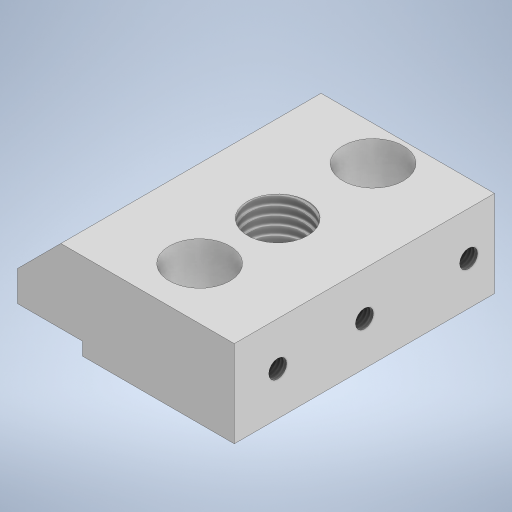
# Autodesk Inventor part: spannbakce
Saved by Autodesk Inventor 2024 (Build 280153000, 153)
## iProperties
Created: 2024-01-30
Part Number: spannbakce
Material: Generisch
Document SubType Name: Modeling
Designer: ffogue
Density: 1 g/cm^3
Appearance: Vorgabe
Author: ffogue
Autodesk Inventor part; units mm, degrees
note: some values were not read from the file. Chosen so that the rebuilt part matches the saved one: direction of "Bohrung2"; direction of "Bohrung3".
ref_plane "YZ Plane" through (0, 0, 0) normal (1, 0, 0) x (0, 1, 0)
ref_plane "XZ Plane" through (0, 0, 0) normal (0, 1, 0) x (-1, 0, 0)
ref_plane "XY Plane" through (0, 0, 0) normal (0, 0, 1) x (1, 0, 0)
sketch "Skizze1" plane through (0, 0, 0) normal (0, 1, 0) x (-1, 0, 0)
  line L0 (0, -10) -> (0, 10)
  line L1 (0, 10) -> (40, 10)
  line L2 (40, 10) -> (50, 0)
  line L3 (50, 0) -> (50, -7)
  line L4 (50, -7) -> (35, -7)
  line L5 (35, -7) -> (35, -10)
  line L6 (35, -10) -> (0, -10)
  line L7 (0, 0) -> (85.3703, 0) construction
  dimension "d0" = 10
  dimension "d1" = 10
  dimension "d2" = 3
  dimension "d3" = 20
  dimension "d4" = 40
  dimension "d5" = 15
  constraints: 17 end point, 5 perpendicular, 1 coincident, 1 horizontal, 1 midpoint, 1 vertical
  measures "d0" horizontal distance of L2.end L1.end
  measures "d1" horizontal distance of L2.end L1.end
  measures "d2" distance between parallel lines of L6 L4
  measures "d3" distance between parallel lines of L6 L1
  measures "d4" distance from line of L0 L1.end
  measures "d5" distance between parallel lines of L5 L3
extrude "Extrusion1" add sketch "Skizze1" along normal blind 60
sketch "Skizze2" plane through (-35, 0, -7) normal (0, 0, -1) x (-1, 0, 0)
  line L0 (15, 0) -> (15, 60) projected
  line L1 (15, 30) -> (5.3736, 30) construction
  line L2 (0, 60) -> (15, 60) projected
  point P0 (-35, 0)
  point P1 (8, 10)
  point P2 (8, 50)
  dimension "d8" = 7
  dimension "d9" = 7
  dimension "d10" = 40
  dimension "d11" = 10
  constraints: 2 end point, 1 horizontal, 1 midpoint
  measures "d8" distance from line of L0 point (8, 10)
  measures "d9" distance from line of point (8, 50) L0
  measures "d10" distance of point (8, 10) point (8, 50)
  measures "d11" distance from line of point (8, 50) L2
hole "Bohrung1" at (-43, 10, -7) at (-43, 50, -7) direction (0, 0, 1) diameter 3.242 depth 12 tip angle 118 thread size "M4x0.7" class "6H" standard "ISO Metric profile"
sketch "Skizze3" plane through (0, 0, -10) normal (0, 0, -1) x (-1, 0, 0)
  line L0 (0, 0) -> (0, 60) projected
  line L1 (0, 0) -> (35, 0) projected
  point P0 (20, 52)
  point P1 (20, 30)
  point P2 (20, 12)
  point P3 (0, 30)
  dimension "d19" = 20
  dimension "d20" = 12
  dimension "d21" = 40
  constraints: 3 vertical alignment, 1 horizontal alignment, 1 midpoint
  measures "d19" distance from line of L0 point (20, 52)
  measures "d20" distance from line of L1 point (20, 12)
  measures "d21" distance of point (20, 12) point (20, 52)
hole "Bohrung2" at (-20, 12, -10) at (-20, 52, -10) direction (0, 0, 1) diameter 14 depth 20
hole "Bohrung3" at (-20, 30, -10) direction (0, 0, 1) diameter 13.835 depth 20 thread size "M16x2" class "6H" standard "ISO Metric profile"
sketch "Skizze6" plane through (0, 0, 10) normal (1, 0, 0) x (0, 0, -1)
  line L0 (0, 60) -> (20, 60) projected
  point P0 (10, 0)
  point P1 (10, 54.0188)
  point P2 (10, 60)
  constraints: 1 midpoint, 1 vertical alignment
hole "Bohrung4" at (0, 54.0188, 0) direction (-1, 0, 0) diameter 4.134 depth 10 tip angle 118 thread size "M5x0.8" class "6H" standard "ISO Metric profile"
sketch "Skizze7" plane through (0, 0, 10) normal (1, 0, 0) x (0, 0, -1)
  line L0 (0, 0) -> (20, 0) projected
  point P0 (10, 0)
  point P1 (10, 10)
  point P2 (10, 0)
  point P3 (10, 0)
  dimension "d51" = 10
  constraints: 2 midpoint, 1 vertical alignment
  measures "d51" distance of point (10, 0) point (10, 10)
hole "Bohrung5" at (0, 10, 0) direction (-1, 0, 0) diameter 4.134 depth 10 tip angle 118 thread size "M5x0.8" class "6H" standard "ISO Metric profile"
sketch "Skizze8" plane through (0, 0, 10) normal (1, 0, 0) x (0, 0, -1)
  line L0 (0, 0) -> (20, 0) projected
  point P0 (10, 0)
  point P1 (10, 30)
  point P2 (10, 0)
  point P3 (10, 0)
  point P4 (10, 0)
  dimension "d59" = 30
  constraints: 3 midpoint, 2 vertical alignment
  measures "d59" distance of point (10, 0) point (10, 30)
hole "Bohrung6" at (0, 30, 0) direction (-1, 0, 0) diameter 4.134 depth 10 tip angle 118 thread size "M5x0.8" class "6H" standard "ISO Metric profile"
